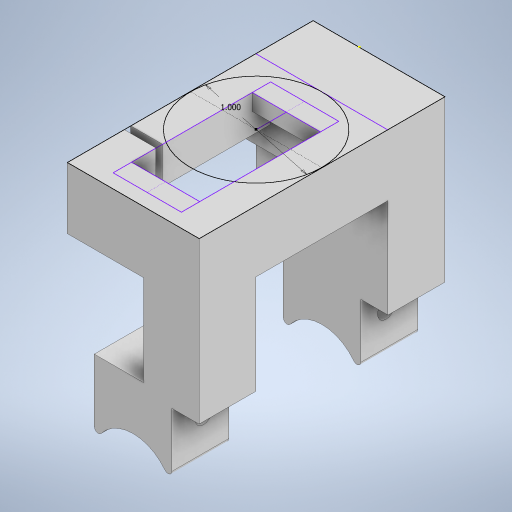
# Autodesk Inventor part: Servo Mount V5
Saved by Autodesk Inventor 2024 (Build 280153000, 153)
## iProperties
Created: 2024-11-24
Part Number: Servo Mount V5
Material: Generic
Document SubType Name: Modeling
Designer: Tommy Rohmann
Density: 1 g/cm^3
Appearance: Default
Author: Tommy Rohmann
Autodesk Inventor part; units mm, degrees
ref_plane "YZ Plane" through (0, 0, 0) normal (1, 0, 0) x (0, 1, 0)
ref_plane "XZ Plane" through (0, 0, 0) normal (0, 1, 0) x (-1, 0, 0)
ref_plane "XY Plane" through (0, 0, 0) normal (0, 0, 1) x (1, 0, 0)
sketch "Side Block" plane through (0, 0, 0) normal (0, 0, 1) x (1, 0, 0)
  line L0 (11.2978, -7.5275) -> (11.2978, -18.0776)
  line L1 (11.2978, -7.5275) -> (16.5429, -7.5275)
  line L2 (16.5429, -7.5275) -> (16.5429, 23.5875)
  line L3 (16.5429, 23.5875) -> (-8.9841, 23.5875)
  line L4 (-8.9841, 23.5875) -> (-8.9841, -7.5275)
  line L5 (-8.9841, -7.5275) -> (-3.739, -7.5275)
  line L6 (-3.739, -18.0776) -> (-3.739, -7.5275)
  arc A0 (9.9308, -18.5408) -> (-2.3719, -18.5408) centre (3.7794, -23.2501) ccw
  arc A1 (-3.739, -18.0776) -> (-2.3719, -18.5408) centre (-2.977, -18.0776) ccw
  arc A2 (9.9308, -18.5408) -> (11.2978, -18.0776) centre (10.5358, -18.0776) ccw
  point P0 (3.7794, -4.0139)
  point P1 (11.2978, -21.382)
  point P2 (-3.739, -21.382)
  dimension "d2" = 31.115
  dimension "d3" = 31.115
  dimension "d4" = 5.2451
  dimension "d5" = 25.527
  dimension "d9" = 15.494
  dimension "d10" = 0.762
  measures "d2" distance between parallel lines of L3 L1
  measures "d3" distance between parallel lines of L3 L5
  measures "d4" distance between parallel lines of L2 L0
  measures "d5" distance between parallel lines of L2 L4
  measures "d9" diameter of A0
  measures "d10" radius of A1
sketch "Motor Containment" plane through (0, 0, 0) normal (0, 0, 1) x (1, 0, 0)
  line L0 (-35.1538, -13.4444) -> (-35.1538, -17.0004) construction
  line L1 (-35.1538, -40.3684) -> (-35.1538, -43.9244) construction
  line L2 (-35.1538, -17.0004) -> (-35.1538, -22.8424)
  line L3 (-41.7578, -43.9244) -> (-28.5498, -43.9244)
  line L4 (-28.5498, -43.9244) -> (-28.5498, -13.4444)
  line L5 (-28.5498, -13.4444) -> (-41.7578, -13.4444)
  line L6 (-41.7578, -13.4444) -> (-41.7578, -43.9244)
  line L7 (-41.7578, -40.3684) -> (-28.5498, -40.3684)
  line L8 (-28.5498, -40.3684) -> (-28.5498, -17.0004)
  line L9 (-28.5498, -17.0004) -> (-41.7578, -17.0004)
  line L10 (-41.7578, -17.0004) -> (-41.7578, -40.3684)
  point P0 (-35.1538, -28.1145)
  dimension "d17" = 13.208
  dimension "d18" = 30.48
  dimension "d19" = 23.368
  dimension "d20" = 5.842
  measures "d17" distance of L5.end L4.end
  measures "d18" distance of L4.end L3.end
  measures "d19" distance of L8.end L7.end
  measures "d20" distance of L0.end L2.end
sketch "Sketch1" plane through (0, 0, 0) normal (0, 0, 1) x (1, 0, 0)
  line L0 (11.2978, -7.5275) -> (11.2978, -18.0776)
  line L1 (11.2978, -7.5275) -> (16.5429, -7.5275)
  line L2 (16.5429, -7.5275) -> (16.5429, 23.5875)
  line L3 (16.5429, 23.5875) -> (-8.9841, 23.5875)
  line L4 (-8.9841, 23.5875) -> (-8.9841, -7.5275)
  line L5 (-8.9841, -7.5275) -> (-3.739, -7.5275)
  line L6 (-3.739, -18.0776) -> (-3.739, -7.5275)
  arc A0 (9.9308, -18.5408) -> (-2.3719, -18.5408) centre (3.7794, -23.2501) ccw
  arc A1 (-3.739, -18.0776) -> (-2.3719, -18.5408) centre (-2.977, -18.0776) ccw
  arc A2 (9.9308, -18.5408) -> (11.2978, -18.0776) centre (10.5358, -18.0776) ccw
  point P0 (0, 0)
  dimension "d6" = 23.5875
extrude "Extrusion1" add sketch "Sketch1" along normal blind 47.5742
sketch "Sketch2" plane through (-8.9841, 23.5875, 0) normal (0, 1, 0) x (1, 0, 0)
  line L0 (0, -47.5742) -> (5.2451, -47.5742) projected
  line L1 (20.2819, 0) -> (25.527, 0) projected
  line L2 (0, -47.5742) -> (25.527, -47.5742)
  line L3 (25.527, -47.5742) -> (25.527, 0)
  line L4 (25.527, 0) -> (0, 0)
  line L5 (0, 0) -> (0, -47.5742)
  line L6 (0, -23.7871) -> (25.527, -23.7871) construction
  circle A0 centre (12.7635, -23.7871) radius 12.7
  line L7 (0, 0) -> (0, -47.5742) projected
  line L8 (0, -11.0871) -> (25.527, -11.0871)
  line L9 (12.7635, -14.3891) -> (12.7635, -17.9451) construction
  line L10 (12.7635, -41.3131) -> (12.7635, -44.8691) construction
  line L11 (12.7635, -17.9451) -> (12.7635, -23.7871)
  line L12 (6.1595, -44.8691) -> (19.3675, -44.8691)
  line L13 (19.3675, -44.8691) -> (19.3675, -14.3891)
  line L14 (19.3675, -14.3891) -> (6.1595, -14.3891)
  line L15 (6.1595, -14.3891) -> (6.1595, -44.8691)
  line L16 (6.1595, -41.3131) -> (19.3675, -41.3131)
  line L17 (19.3675, -41.3131) -> (19.3675, -17.9451)
  line L18 (19.3675, -17.9451) -> (6.1595, -17.9451)
  line L19 (6.1595, -17.9451) -> (6.1595, -41.3131)
  point P0 (8.9841, 0)
  point P1 (6.1595, -17.9451)
  dimension "d21" = 25.4
  constraints: 12 end point, 2 horizontal, 2 midpoint, 2 parallel, 2 perpendicular, 2 point on line, 1 centre point, 1 other
  measures "d21" diameter of A0
sketch "Sketch3" plane through (-8.9841, -7.5275, 0) normal (-1, 0, 0) x (0, 0, 1)
  line L0 (0, 19.177) -> (47.5742, 19.177)
  line L1 (47.5742, 31.115) -> (47.5742, 0) projected
  line L2 (0, 31.115) -> (47.5742, 31.115) projected
  line L3 (41.4528, 31.115) -> (41.4528, -19.3537) construction
  line L4 (6.1214, 31.115) -> (6.1214, -20.7554) construction
  line L5 (0, 31.115) -> (0, 0) construction
  circle A0 centre (6.1214, -4.1148) radius 1.6637
  circle A1 centre (41.4528, -4.1148) radius 1.6637
  line L6 (23.7871, 31.115) -> (23.7871, -19.3537) construction
  line L7 (36.576, 19.177) -> (36.576, -23.6144)
  line L8 (10.9982, 19.177) -> (10.9982, -23.6144)
  line L9 (36.576, -23.6144) -> (10.9982, -23.6144)
  line L10 (0, 0) -> (47.5742, 0) projected
  point P0 (10.9982, 19.177)
  dimension "d26" = 11.938
  dimension "d27" = 6.1214
  dimension "d28" = 6.1214
  dimension "d29" = 3.3274
  dimension "d30" = 3.3274
  dimension "d33" = 10.9982
  dimension "d54" = 4.1148
  dimension "d55" = 4.1148
  constraints: 14 end point, 6 point on line, 4 vertical, 2 centre point, 2 horizontal, 2 symmetric about line, 1 midpoint
  measures "d26" distance between parallel lines of L2 L0
  measures "d27" distance between parallel lines of L5 L4
  measures "d28" distance between parallel lines of L1 L3
  measures "d29" diameter of A0
  measures "d30" diameter of A1
  measures "d33" distance between parallel lines of L1 L7
  measures "d54" distance from line of L10 A0.centre
  measures "d55" distance from line of L10 A1.centre
extrude "Extrusion4" cut sketch "Sketch3" against normal blind 46.0375 contours L0 L7 L10 L8 | L10 L7 L9 L8 | A0 | A1
extrude "Extrusion5" cut sketch "Sketch2" against normal blind 23.8125 contours L15 L18 L13 A0 | A0 L13 L16 L15 | L15 L14 L13 L18 | L16 L13 L12 L15
sketch "Sketch4" plane through (0, 0, 47.5742) normal (0, 0, 1) x (1, 0, 0)
  line L0 (16.5429, 23.5875) -> (-8.9841, 23.5875) construction
  line L1 (3.7794, 23.5875) -> (3.7794, -25.467) construction
  line L2 (5.8114, 11.6495) -> (5.8114, -5.94)
  line L3 (-8.9841, 11.6495) -> (-8.9841, -7.5275) projected
  line L4 (-8.9841, -5.94) -> (16.5429, -5.94)
  line L5 (16.5429, -7.5275) -> (16.5429, 11.6495) projected
  line L6 (-8.9841, -7.5275) -> (-3.739, -7.5275) projected
  line L7 (-8.9841, 11.6495) -> (-2.8246, 11.6495) projected
  line L8 (-8.9841, 11.6495) -> (5.8114, 11.6495)
  line L9 (-3.739, -7.5275) -> (-3.739, -18.0776) projected
  line L10 (-3.739, -7.5275) -> (-3.739, -5.94)
  point P0 (0, 0)
  dimension "d38" = 2.032
  dimension "d39" = 1.5875
  constraints: 10 end point, 4 point on line, 2 perpendicular, 2 vertical, 1 horizontal, 1 midpoint
  measures "d38" distance between parallel lines of L1 L2
  measures "d39" distance between parallel lines of L4 L6
extrude "Extrusion6" cut sketch "Sketch4" against normal blind 14.2875
chamfer "Chamfer1" distance 4.7625 angle 45 1 edges at (-2.8246, 11.6495, 29.6291)
sketch "Sketch5" plane through (3.7794, -23.2501, 36.576) normal (0, 0, -1) x (-1, 0, 0)
  line L0 (-6.604, 23.0251) -> (-6.604, 34.8996) projected
  line L1 (-6.604, 23.0251) -> (-2.032, 18.4531)
  line L2 (-2.032, 17.3101) -> (-2.032, 23.0251) projected
  line L3 (-6.604, 23.0251) -> (-0.1382, 23.0251) construction
  line L4 (-2.032, 18.4531) -> (-2.032, 23.0251)
  line L5 (-2.032, 23.0251) -> (-6.604, 23.0251)
  point P0 (3.7794, 23.2501)
  dimension "d45" = 45
  constraints: 8 end point, 1 collinear, 1 equal length, 1 horizontal, 1 perpendicular, 1 point on line
  measures "d45" angle of L1 L3
extrude "Extrusion7" cut sketch "Sketch5" against normal up to surface (8.2931 mm away)
extrude "Extrusion8" add sketch "Sketch2" against normal blind 3.175 contours L15 L14 L13 L18 | L16 L13 L12 L15
sketch "Sketch6" plane through (-8.9841, -7.5275, 0) normal (-1, 0, 0) x (0, 0, 1)
  line L0 (0, 31.115) -> (47.5742, 31.115) projected
  line L1 (36.576, 19.177) -> (14.3891, 19.177) projected
  line L2 (36.576, 31.115) -> (35.306, 31.115)
  line L3 (35.306, 31.115) -> (35.306, 19.177)
  line L4 (35.306, 19.177) -> (36.576, 19.177)
  line L5 (36.576, 19.177) -> (36.576, 31.115)
  line L6 (36.576, 7.3025) -> (36.576, 19.177) projected
  point P0 (0, 7.5275)
  dimension "d52" = 0
  dimension "d53" = 1.27
  constraints: 8 end point, 2 parallel, 2 point on line, 1 horizontal, 1 perpendicular
  measures "d52" distance between parallel lines of L6 L5
  measures "d53" distance between parallel lines of L5 L3
extrude "Extrusion9" cut sketch "Sketch6" against normal blind 14.2875
equation "\"d27\" = d28"
equation "\"d30\" = d29"
body "Solid1"
